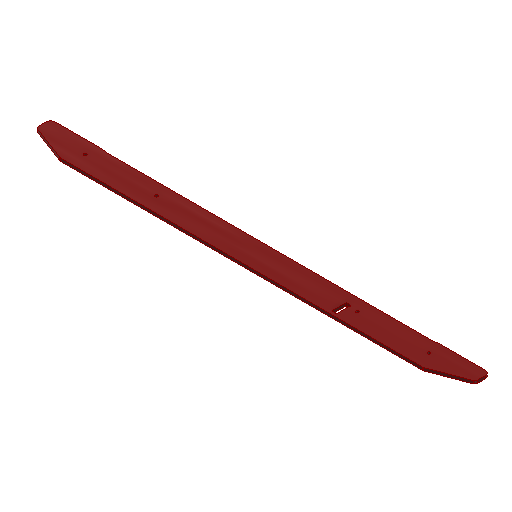
# Autodesk Inventor part: LC_PLEXI_3mm_Heatbed_Platform_Logo_Plate_Diffuser
Saved by Autodesk Inventor 2026.1 (Build 301233000, 233)
## iProperties
Created: 2016-06-27
Part Number: LC_PLEXI_3mm_Heatbed_Platform_Logo_Plate_Diffuser
Material: Ogólny
Document SubType Name: Modeling
Designer: Andrzej
Density: 1 g/cm^3
Appearance: Odbijająca — czerwona
Author: Andrzej
Autodesk Inventor part; units mm, degrees
ref_plane "YZ Plane" through (0, 0, 0) normal (1, 0, 0) x (0, 1, 0)
ref_plane "XZ Plane" through (0, 0, 0) normal (0, 1, 0) x (-1, 0, 0)
ref_plane "XY Plane" through (0, 0, 0) normal (0, 0, 1) x (1, 0, 0)
sketch "Szkic1" plane through (0, 0, 0) normal (0, 0, 1) x (1, 0, 0)
  line L0 (444.7232, 18.712) -> (444.7232, -11.288)
  line L1 (444.7232, -11.288) -> (-15.2768, -11.288)
  line L2 (-15.2768, -11.288) -> (-15.2768, 18.712)
  line L3 (-15.2768, 18.712) -> (36.1232, 18.712)
  line L4 (36.1232, 18.712) -> (36.1232, 17.712)
  line L5 (36.1232, 17.712) -> (393.3232, 17.712)
  line L6 (393.3232, 17.712) -> (393.3232, 18.712)
  line L7 (393.3232, 18.712) -> (444.7232, 18.712)
  point P0 (0, 0)
  dimension "d0" = 460
  dimension "d1" = 30
  dimension "d2" = 1
  dimension "d3" = 51.4
  dimension "d4" = 51.4
  constraints: 16 end point, 4 perpendicular, 1 horizontal, 1 parallel, 1 point on line
  measures "d0" distance of L0.end L1.end
  measures "d1" distance of L0.start L0.end
  measures "d2" distance between parallel lines of L3 L5
  measures "d3" distance of L2.end L3.end
  measures "d4" distance of L6.end L0.start
extrude "Wyciągnięcie proste1" add sketch "Szkic1" along normal blind 3
chamfer "Faza1" distance 10 distance2 1 1 edges at (36.1232, 17.712, 1.5) measured on face at (274.2565, 17.712, 1)
chamfer "Faza2" distance 10 distance2 1 1 edges at (393.3232, 17.712, 1.5) measured on face at (277.5897, 17.712, 1)
fillet "Zaokrąglenie1" radius 5 2 edges at (444.7232, 18.712, 1.5) (-15.2768, 18.712, 1.5)
chamfer "Faza3" distance 40 distance2 15 1 edges at (444.7232, -11.288, 1.5) measured on face at (138.0565, -11.288, 1)
chamfer "Faza4" distance 40 distance2 15 1 edges at (-15.2768, -11.288, 1.5) measured on face at (124.7232, -11.288, 2)
sketch "Szkic2" plane through (0, 0, 3) normal (0, 0, 1) x (1, 0, 0)
  line L0 (383.3232, 17.712) -> (46.1232, 17.712) projected
  line L1 (-15.2768, 13.712) -> (-15.2768, 3.712) projected
  line L2 (444.7232, 3.712) -> (444.7232, 13.712) projected
  line L3 (36.1232, 18.712) -> (-10.2768, 18.712) projected
  line L4 (439.7232, 18.712) -> (393.3232, 18.712) projected
  point P0 (0, 0)
  point P1 (34.7232, 4.712)
  point P2 (394.7232, 4.712)
  point P3 (109.7232, 4.712)
  point P4 (319.7232, 4.712)
  dimension "d34" = 50
  dimension "d35" = 75
  dimension "d36" = 75
  dimension "d37" = 50
  dimension "d39" = 14
  dimension "d40" = 14
  dimension "d41" = 14
  dimension "d42" = 14
  measures "d34" distance from line of point (34.723, 4.712) L1
  measures "d35" distance of point (34.723, 4.712) point (109.723, 4.712)
  measures "d36" distance of point (394.723, 4.712) point (319.723, 4.712)
  measures "d37" distance from line of L2 point (394.723, 4.712)
  measures "d39" distance from line of point (34.723, 4.712) L3
  measures "d40" distance from line of L3 point (109.723, 4.712)
  measures "d41" distance from line of L4 point (319.723, 4.712)
  measures "d42" distance from line of L4 point (394.723, 4.712)
fillet "Zaokrąglenie2" radius 3 4 edges at (444.7232, 3.712, 1.5) (404.7232, -11.288, 1.5) (24.7232, -11.288, 1.5) (-15.2768, 3.712, 1.5)
hole "Otwór1" at (34.7232, 4.712, 3) at (394.7232, 4.712, 3) at (109.7232, 4.712, 3) at (319.7232, 4.712, 3) direction (0, 0, -1) diameter 3 end through all
sketch "Szkic4" plane through (0, 0, 0) normal (0, 0, -1) x (-1, 0, 0)
  circle A0 centre (-109.7232, 4.712) radius 1.5 projected
  circle A1 centre (-34.7232, 4.712) radius 1.5 projected
  circle A2 centre (-394.7232, 4.712) radius 1.5 projected
  circle A3 centre (-319.7232, 4.712) radius 1.5 projected
  arc A4 (13.3302, 2.9821) -> (15.2768, 5.791) centre (12.2768, 5.791) ccw projected
  line L0 (15.2768, 13.712) -> (15.2768, 5.791) projected
  arc A5 (15.2768, 13.712) -> (10.2768, 18.712) centre (10.2768, 13.712) ccw projected
  line L1 (-36.1232, 18.712) -> (10.2768, 18.712) projected
  line L2 (-46.1232, 17.712) -> (-36.1232, 18.712) projected
  line L3 (-383.3232, 17.712) -> (-46.1232, 17.712) projected
  line L4 (-393.3232, 18.712) -> (-383.3232, 17.712) projected
  line L5 (-439.7232, 18.712) -> (-393.3232, 18.712) projected
  arc A6 (-439.7232, 18.712) -> (-444.7232, 13.712) centre (-439.7232, 13.712) ccw projected
  line L6 (-444.7232, 5.791) -> (-444.7232, 13.712) projected
  arc A7 (-444.7232, 5.791) -> (-442.7766, 2.9821) centre (-441.7232, 5.791) ccw projected
  line L7 (-405.2326, -11.0969) -> (-442.7766, 2.9821) projected
  arc A8 (-405.2326, -11.0969) -> (-404.1792, -11.288) centre (-404.1792, -8.288) ccw projected
  line L8 (-25.2672, -11.288) -> (-404.1792, -11.288) projected
  arc A9 (-25.2672, -11.288) -> (-24.2138, -11.0969) centre (-25.2672, -8.288) ccw projected
  line L9 (13.3302, 2.9821) -> (-24.2138, -11.0969) projected
  line L10 (-292.2232, 13.612) -> (-12.8371, 13.612) construction
  line L11 (-12.8371, 13.612) -> (-12.8371, -7.1032) construction
  line L12 (-12.8371, -7.1032) -> (-292.2232, -7.1032) construction
  line L13 (-292.2232, -7.1032) -> (-292.2232, 13.612) construction
  point P0 (0, 0)
  dimension "d43" = 4.1
  dimension "d44" = 152.5
  constraints: 2 other
  measures "d43" distance between parallel lines of L3 L10
  measures "d44" distance between parallel lines of L6 L13
extrude "Wyciągnięcie proste3" [suppressed]
sketch "Szkic5" plane through (0, 0, 0) normal (0, 0, -1) x (-1, 0, 0)
  arc A0 (13.3302, 2.9821) -> (15.2768, 5.791) centre (12.2768, 5.791) ccw projected
  line L0 (15.2768, 13.712) -> (15.2768, 5.791) projected
  arc A1 (15.2768, 13.712) -> (10.2768, 18.712) centre (10.2768, 13.712) ccw projected
  line L1 (-36.1232, 18.712) -> (10.2768, 18.712) projected
  line L2 (-46.1232, 17.712) -> (-36.1232, 18.712) projected
  line L3 (-383.3232, 17.712) -> (-46.1232, 17.712) projected
  line L4 (-393.3232, 18.712) -> (-383.3232, 17.712) projected
  line L5 (-439.7232, 18.712) -> (-393.3232, 18.712) projected
  arc A2 (-439.7232, 18.712) -> (-444.7232, 13.712) centre (-439.7232, 13.712) ccw projected
  line L6 (-444.7232, 5.791) -> (-444.7232, 13.712) projected
  arc A3 (-444.7232, 5.791) -> (-442.7766, 2.9821) centre (-441.7232, 5.791) ccw projected
  line L7 (-405.2326, -11.0969) -> (-442.7766, 2.9821) projected
  arc A4 (-405.2326, -11.0969) -> (-404.1792, -11.288) centre (-404.1792, -8.288) ccw projected
  line L8 (-25.2672, -11.288) -> (-404.1792, -11.288) projected
  arc A5 (-25.2672, -11.288) -> (-24.2138, -11.0969) centre (-25.2672, -8.288) ccw projected
  line L9 (13.3302, 2.9821) -> (-24.2138, -11.0969) projected
  circle A6 centre (-319.7232, 4.712) radius 1.5 projected
  circle A7 centre (-394.7232, 4.712) radius 1.5 projected
  circle A8 centre (-34.7232, 4.712) radius 1.5 projected
  circle A9 centre (-109.7232, 4.712) radius 1.5 projected
  line L10 (-436.9348, 14.712) -> (34.576, 14.712)
  line L11 (-429.8152, 7.212) -> (-144.7013, 7.212)
  line L12 (-310.7232, 7.212) -> (-305.7232, 7.212)
  line L13 (-305.7232, 7.212) -> (-305.7232, -7.788)
  line L14 (-305.7232, -7.788) -> (-310.7232, -7.788)
  line L15 (-310.7232, -7.788) -> (-310.7232, 7.212)
  line L16 (-428.7978, 2.212) -> (-310.7232, 2.212)
  line L17 (-305.7232, 2.212) -> (-143.684, 2.212)
  line L18 (-434.2328, -5.288) -> (-310.7232, -5.288)
  line L19 (-305.7232, -5.288) -> (47.3582, -5.288)
  point P0 (0, 0)
  dimension "d47" = 3
  dimension "d49" = 2.5
  dimension "d51" = 5
  dimension "d52" = 15
  dimension "d54" = 9
  constraints: 20 end point, 7 horizontal, 5 point on line, 2 parallel, 1 perpendicular
  measures "d47" distance between parallel lines of L3 L10
  measures "d49" distance from line of L11 A6.centre
  measures "d51" distance of L13.end L14.end
  measures "d52" distance of L12.end L13.end
  measures "d54" distance from line of A6.centre L15
extrude "Wyciągnięcie proste4" cut sketch "Szkic5" against normal through all contours L13 L14 L15 L11
fillet "Zaokrąglenie3" radius 1 4 edges at (305.7232, -7.788, 1.5) (310.7232, -7.788, 1.5) (310.7232, 7.212, 1.5) (305.7232, 7.212, 1.5)
equation "\"d4\" = d3"
equation "\"d37\" = d34"
equation "\"d40\" = d39"
equation "\"d41\" = d39"
equation "\"d42\" = d39"
